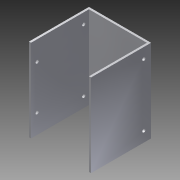
# Autodesk Inventor part: Square pillar
Saved by Autodesk Inventor 2015 (Build 190159000, 159)
## iProperties
Created: 2015-05-26
Part Number: Square pillar
Material: アルミニウム 6061
Document SubType Name: Modeling
Designer: kenta
Density: 2.7 g/cm^3
Appearance: アルミニウム - フラット - Version 1.1
Mass: 74.0434 g
Surface Area: 285.521 cm^2
Volume: 27.4235 cm^3
Author: kenta
Autodesk Inventor part; units mm, degrees
ref_plane "YZ Plane" through (0, 0, 0) normal (1, 0, 0) x (0, 1, 0)
ref_plane "XZ Plane" through (0, 0, 0) normal (0, 1, 0) x (-1, 0, 0)
ref_plane "XY Plane" through (0, 0, 0) normal (0, 0, 1) x (1, 0, 0)
sketch "スケッチ1" plane through (0, 0, 0) normal (0, 0, 1) x (1, 0, 0)
  line L0 (-30, 30) -> (30, 30)
  line L1 (30, 30) -> (30, -30)
  line L2 (30, -30) -> (-30, -30)
  line L3 (-30, -30) -> (-30, 30)
  line L4 (-30, 30) -> (30, -30) construction
  line L5 (30, 30) -> (-30, -30) construction
  line L6 (-28, 28) -> (28, 28)
  line L7 (28, 28) -> (28, -28)
  line L8 (28, -28) -> (-28, -28)
  line L9 (-28, -28) -> (-28, 28)
  line L10 (-28, 28) -> (28, -28) construction
  line L11 (28, 28) -> (-28, -28) construction
  point P0 (0, 0)
  dimension "d0" = 60
  dimension "d1" = 60
  dimension "d2" = 56
  dimension "d3" = 56
  constraints: 24 end point, 4 midpoint, 4 parallel, 2 horizontal, 2 perpendicular
  measures "d0" distance of L1.end L2.end
  measures "d1" distance of L0.end L1.end
  measures "d2" distance of L7.end L8.end
  measures "d3" distance of L6.end L7.end
extrude "押し出し1" add sketch "スケッチ1" along normal blind 80
sketch "スケッチ2" plane through (0, 0, 80) normal (0, 0, 1) x (1, 0, 0)
  line L0 (30, 30) -> (30, -30) projected
  line L1 (-30, -30) -> (30, -30)
  line L2 (30, -30) -> (30, -28)
  line L3 (30, -28) -> (-30, -28)
  line L4 (-30, -28) -> (-30, -30)
  point P0 (0, 0)
  dimension "d6" = 2
  constraints: 8 end point, 2 parallel, 1 horizontal, 1 perpendicular, 1 point on line
  measures "d6" distance of L2.end L1.end
extrude "押し出し2" cut sketch "スケッチ2" against normal blind 100
sketch "スケッチ3" plane through (30, 30, 80) normal (1, 0, 0) x (0, 0, -1)
  line L0 (0, -58) -> (0, 0) projected
  line L1 (80, 0) -> (80, -58) projected
  line L2 (80, 0) -> (0, 0) projected
  point P0 (80, -30)
  point P1 (10, -7)
  point P2 (70, -7)
  dimension "d9" = 60
  dimension "d10" = 10
  dimension "d11" = 10
  dimension "d12" = 7
  dimension "d13" = 7
  measures "d9" distance of point (70, -7) point (10, -7)
  measures "d10" distance from line of L0 point (10, -7)
  measures "d11" distance from line of L1 point (70, -7)
  measures "d12" distance from line of point (10, -7) L2
  measures "d13" distance from line of point (70, -7) L2
hole "穴1" at (30, 23, 70) at (30, 23, 10) direction (-1, 0, 0) diameter 3.2 end through all
sketch "スケッチ4" plane through (-30, 30, 0) normal (-1, 0, 0) x (0, 0, 1)
  line L0 (0, 0) -> (80, 0) projected
  line L1 (80, 0) -> (80, -58) projected
  point P0 (0, -30)
  point P1 (61.25, -52)
  point P2 (18.75, -52)
  dimension "d21" = 52
  dimension "d22" = 42.5
  dimension "d23" = 18.75
  constraints: 1 horizontal alignment
  measures "d21" distance from line of L0 point (61.25, -52)
  measures "d22" distance of point (18.75, -52) point (61.25, -52)
  measures "d23" distance from line of L1 point (61.25, -52)
hole "穴2" at (-30, -22, 61.25) at (-30, -22, 18.75) direction (1, 0, 0) diameter 3.2 depth 8 tip angle 118
